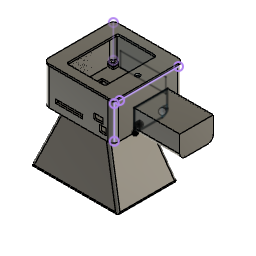
modelofinal (Autodesk Fusion 360 design; units mm, degrees)
Autodesk Fusion 360 part; units mm, degrees
(part 1 of 3)
sketch "Boceto1" plane through (0, 0, 0) normal (0, 0, 1) x (1, 0, 0)
  line L0 (0, 0) -> (95, 0)
  line L1 (95, 0) -> (95, 65)
  line L2 (95, 65) -> (0, 65)
  line L3 (0, 65) -> (0, 0)
  dimension "d1" = 95
  dimension "d2" = 65
  constraint horizontal L0
  constraint vertical L1
  constraint horizontal L2
  constraint vertical L3
  constraint coincident L0.start L3.end
  measures "d1" distance of L1.end L2.end
  measures "d2" distance of L0.start L2.end
extrude "Extruir1" add sketch "Boceto1" along normal blind 1.5 makes body 1
sketch "Boceto3" plane through (47.5, 32.5, 66.5) normal (0, 0, 1) x (1, 0, 0)
  line L0 (-47.5, 32.5) -> (-47.5, -32.5)
  line L1 (-47.5, -32.5) -> (47.5, -32.5)
  line L2 (47.5, -32.5) -> (47.5, 32.5)
  line L3 (47.5, 32.5) -> (-47.5, 32.5)
  line L4 (-22.128, 7.128) -> (-22.128, -7.128) construction
  line L5 (-22.128, -7.128) -> (22.128, -7.128) construction
  line L6 (22.128, -7.128) -> (22.128, 7.128) construction
  line L7 (22.128, 7.128) -> (-22.128, 7.128) construction
  line L8 (22.5, 20) -> (-22.5, 20)
  line L9 (-22.5, 20) -> (-22.5, -20)
  line L10 (-22.5, -20) -> (22.5, -20)
  line L11 (22.5, -20) -> (22.5, 20)
  dimension "d11" = -25.372
  dimension "d12" = 45
  dimension "d13" = 40
  dimension "d14" = 12.5
  dimension "d15" = 25
  constraint horizontal L8
  constraint vertical L9
  constraint horizontal L10
  constraint vertical L11
  measures "d12" distance of L8.start L8.end
  measures "d13" distance of L8.start L10.end
  measures "d14" distance of L3 L8
  measures "d15" distance of L0 L9
loft "Solevación1" add profiles "Boceto3" section 1 face at (31.6667, 43.3333, 1.5) section 2 contours L8 L9 L10 L11 on bodies 1 bodies 1
shell "Vaciado1" thickness 2 removed faces 1 at (40, 25.8333, 66.5) on bodies 1
extrude "Extruir2" add 1 faces at (25.7143, 26.5122, 66.5) along direction (0, 0, 1) blind 5 on bodies 1 bodies 1
sketch "Boceto4" plane through (25, 0, 0) normal (-1, 0, 0) x (0, -1, 0)
  line L0 (-52.5, 66.5) -> (-12.5, 66.5)
  line L1 (-12.5, 66.5) -> (-12.5, 71.5)
  line L2 (-12.5, 71.5) -> (-52.5, 71.5)
  line L3 (-52.5, 71.5) -> (-52.5, 66.5)
  circle A0 centre (-46.5, 69) radius 1.5
  circle A1 centre (-18.5, 69) radius 1.5
  dimension "d19" = 3
  dimension "d20" = 6
  dimension "d21" = 3
  dimension "d22" = 6
  measures "d19" diameter of A0
  measures "d20" distance of L3 A0.centre
  measures "d21" diameter of A1
  measures "d22" distance of L1 A1.centre
extrude "Extruir3" cut sketch "Boceto4" against normal blind 50 contours A0 | A1 bodies 1
sketch "Boceto5" plane through (-0.5026, 0, 0.1933) normal (-0.933346, 0, 0.358979) x (0, -1, 0)
  line L0 (-65, 1.4) -> (0, 1.4)
  line L1 (0, 1.4) -> (-12.5, 71.042)
  line L2 (-12.5, 71.042) -> (-52.5, 71.042)
  line L3 (-63.6538, 8.9) -> (-1.3462, 8.9)
  line L4 (-62.968, 1.4) -> (-61.6219, 8.9)
  line L5 (-2.032, 1.4) -> (-3.3781, 8.9)
  line L6 (-65, 1.4) -> (-52.5, 71.042)
  dimension "d27" = 2
  dimension "d28" = 2
  constraint coincident L1 L3.end
  constraint horizontal L3
  constraint coincident L0 L4.start
  constraint coincident L3 L4.end
  constraint coincident L0 L5.start
  constraint coincident L3 L5.end
  constraint parallel L4 L6
  constraint parallel L1 L5
  measures "d27" distance of L1 L5
  measures "d28" distance of L4 L6
extrude "Extruir4" cut sketch "Boceto5" against normal blind 1 contours L0 L3 L4 L5 bodies 1
fillet "Empalme1" radius 2.5 4 edges at (82.5, 6.25, 34) (12.5, 6.25, 34) (82.5, 58.75, 34) (12.5, 58.75, 34) on bodies 1
extrude "Extruir5" cut 1 faces at (1.8308, 22.7927, 3.4744) along direction (0.933346, 0, -0.358979) blind 1 on bodies 1 bodies 1
sketch "Boceto6" plane through (0, 0, 71.5) normal (0, 0, 1) x (-1, 0, 0)
  line L0 (-27.1428, -50.4634) -> (-67.8572, -50.4634)
  line L1 (-67.8572, -50.4634) -> (-67.8572, -14.5366)
  line L2 (-67.8572, -14.5366) -> (-27.1428, -14.5366)
  line L3 (-27.1428, -14.5366) -> (-27.1428, -50.4634)
  line L4 (-70, -52.5) -> (-25, -52.5)
  line L5 (-25, -52.5) -> (-25, -12.5)
  line L6 (-25, -12.5) -> (-70, -12.5)
  line L7 (-70, -12.5) -> (-70, -52.5)
sketch "Boceto7" plane through (47.5, 32.5, 71.51) normal (0, 0, 1) x (1, 0, 0)
sketch "Boceto8" plane through (0, 0, 71.5) normal (0, 0, 1) x (1, 0, 0)
sketch "Boceto9" plane through (0, 0, 71.5) normal (0, 0, 1) x (1, 0, 0)
  line L0 (27.1833, 50.4311) -> (67.8663, 50.4311)
  line L1 (67.8663, 50.4311) -> (67.8663, 14.5442)
  line L2 (67.8663, 14.5442) -> (27.1833, 14.5442)
  line L3 (27.1833, 14.5442) -> (27.1833, 50.4311)
  constraint horizontal L0
  constraint vertical L1
  constraint horizontal L2
  constraint vertical L3
ref_plane "PlanoDeObra3" through (47.5, 32.5, 71.6) normal (0, 0, 1) x (-1, 0, 0)
sketch "Boceto10" plane through (0, 0, 71.5) normal (0, 0, 1) x (-1, 0, 0)
  line L0 (-27.2, -50.4) -> (-67.7844, -50.4)
  line L1 (-67.7844, -50.4) -> (-67.7844, -14.5685)
  line L2 (-67.7844, -14.5685) -> (-27.2, -14.5685)
  line L3 (-27.2, -14.5685) -> (-27.2, -50.4)
  line L4 (-29.2, -16.5685) -> (-29.2, -48.4)
  line L5 (-29.2, -48.4) -> (-65.7844, -48.4)
  line L6 (-65.7844, -48.4) -> (-65.7844, -16.5685)
  line L7 (-65.7844, -16.5685) -> (-29.2, -16.5685)
  dimension "d37" = 2
  constraint horizontal L0
  constraint vertical L1
  constraint horizontal L2
  constraint vertical L3
extrude "Extruir6" add sketch "Boceto10" against normal blind 5 separate body makes body 2
sketch "Boceto11" plane through (0, 0, 71.5) normal (0, 0, 1) x (1, 0, 0)
sketch "Boceto12" plane through (0, 0, 71.5) normal (0, 0, 1) x (1, 0, 0)
  line L0 (90.1428, -5.0366) -> (25.1428, -5.0366)
  line L1 (20.1428, -0.0366) -> (20.1428, 64.9634)
  line L2 (25.1428, 69.9634) -> (90.1428, 69.9634)
  line L3 (95.1428, 64.9634) -> (95.1428, -0.0366)
  line L4 (65.8572, 16.5366) -> (29.1428, 16.5366)
  line L5 (29.1428, 16.5366) -> (29.1428, 48.4634)
  line L6 (29.1428, 48.4634) -> (65.8572, 48.4634)
  line L7 (65.8572, 48.4634) -> (65.8572, 16.5366)
  line L8 (27.1428, 50.4634) -> (67.8572, 50.4634)
  line L9 (27.1428, 14.5366) -> (27.1428, 50.4634)
  line L10 (67.8572, 14.5366) -> (27.1428, 14.5366)
  line L11 (67.8572, 50.4634) -> (67.8572, 14.5366)
  circle A0 centre (91.1428, 65.9634) radius 1.5
  circle A1 centre (24.1428, 65.9634) radius 1.5
  circle A2 centre (91.1428, -1.0366) radius 1.5
  arc A3 (90.1428, -5.0366) -> (95.1428, -0.0366) centre (90.1428, -0.0366) ccw
  circle A4 centre (24.1428, -2.0366) radius 1.5
  arc A5 (20.1428, -0.0366) -> (25.1428, -5.0366) centre (25.1428, -0.0366) ccw
  arc A6 (95.1428, 64.9634) -> (90.1428, 69.9634) centre (90.1428, 64.9634) ccw
  arc A7 (25.1428, 69.9634) -> (20.1428, 64.9634) centre (25.1428, 64.9634) ccw
  point P0 (95.1428, -5.0366)
  point P1 (20.1428, -5.0366)
  point P2 (20.1428, 69.9634)
  dimension "d40" = 2
  dimension "d41" = 2
  dimension "d42" = 2
  dimension "d43" = 2
  dimension "d44" = 75
  dimension "d45" = 75
  dimension "d46" = 9
  dimension "d47" = 19.5
  dimension "d48" = 3
  dimension "d49" = 4
  dimension "d50" = 4
  dimension "d51" = 3
  dimension "d52" = 4
  dimension "d53" = 4
  dimension "d54" = 5
  dimension "d55" = 4
  dimension "d56" = 4
  dimension "d57" = 3
  dimension "d58" = 3
  dimension "d59" = 3
  dimension "d60" = 4
  dimension "d61" = 5
  dimension "d62" = 5
  dimension "d63" = 5
  constraint horizontal L0
  constraint vertical L1
  constraint horizontal L2
  constraint vertical L3
  constraint horizontal L4
  constraint vertical L5
  constraint horizontal L6
  constraint vertical L7
  constraint coincident P0 L0
  constraint coincident P0 L3
  constraint tangent L0 A3
  constraint tangent L3 A3
  constraint coincident P1 L0
  constraint coincident P1 L1
  constraint tangent L0 A5
  constraint tangent L1 A5
  constraint tangent L2 A6
  constraint tangent L3 A6
  constraint coincident P2 L1
  constraint coincident P2 L2
  constraint tangent L1 A7
  constraint tangent L2 A7
  measures "d40" distance of L6 L8
  measures "d41" distance of L5 L9
  measures "d42" distance of L4 L10
  measures "d43" distance of L7 L11
  measures "d44" distance of P1 P2
  measures "d45" distance of P0 P1
  measures "d46" distance of L1 L5
  measures "d47" distance of L2 L8
  measures "d48" diameter of A0
  measures "d49" distance of L2 A0.centre
  measures "d50" distance of L3 A0.centre
  measures "d51" diameter of A2
  measures "d52" distance of L3 A2.centre
  measures "d53" distance of L0 A2.centre
  measures "d54" radius of A3
  measures "d55" distance of L2 A1.centre
  measures "d56" distance of L1 A1.centre
  measures "d57" diameter of A1
  measures "d58" diameter of A4
  measures "d59" distance of L0 A4.centre
  measures "d60" distance of L1 A4.centre
  measures "d61" radius of A5
  measures "d62" radius of A6
  measures "d63" radius of A7
extrude "Extruir7" add sketch "Boceto12" along normal blind 2 contours L0 L1 L2 L3 A3 A5 A6 A7 | L8 L9 L10 L11 bodies 2
sketch "Boceto13" plane through (0, 0, 71.5) normal (0, 0, -1) x (1, 0, 0)
  arc A0 (90.1428, -69.9634) -> (95.1428, -64.9634) centre (90.1428, -64.9634) ccw
  line L0 (95.1428, -64.9634) -> (95.1428, 0.0366)
  arc A1 (95.1428, 0.0366) -> (90.1428, 5.0366) centre (90.1428, 0.0366) ccw
  line L1 (90.1428, 5.0366) -> (25.1428, 5.0366)
  arc A2 (25.1428, 5.0366) -> (20.1428, 0.0366) centre (25.1428, 0.0366) ccw
  line L2 (20.1428, 0.0366) -> (20.1428, -64.9634)
  arc A3 (20.1428, -64.9634) -> (25.1428, -69.9634) centre (25.1428, -64.9634) ccw
  line L3 (25.1428, -69.9634) -> (90.1428, -69.9634)
  circle A4 centre (91.1428, -65.9634) radius 1.5
  circle A5 centre (24.1428, -65.9634) radius 1.5
  circle A6 centre (91.1428, 1.0366) radius 1.5
  circle A7 centre (24.1428, 2.0366) radius 1.5
  line L4 (67.7844, -14.5685) -> (67.7844, -50.4)
  line L5 (67.7844, -50.4) -> (27.2, -50.4)
  line L6 (27.2, -50.4) -> (27.2, -14.5685)
  line L7 (27.2, -14.5685) -> (67.7844, -14.5685)
  circle A8 centre (24.1428, 2.0366) radius 1.5
  circle A9 centre (91.1428, 1.0366) radius 1.5
  circle A10 centre (91.1428, -65.9634) radius 1.5
  circle A11 centre (24.1428, -65.9634) radius 1.5
  constraint concentric A7 A8
  constraint concentric A6 A9
  constraint concentric A4 A10
  constraint concentric A5 A11
extrude "Extruir8" add sketch "Boceto13" against normal blind 1 contours A4 A10 | A5 A11 | A6 A9 | A7 A8 bodies 2
sketch "Boceto14" plane through (25, 0, 0) normal (-1, 0, 0) x (0, -1, 0)
  circle A0 centre (-18.5, 69) radius 1.5
  circle A1 centre (-46.5, 69) radius 1.5
  line L0 (-12.5, 63.9895) -> (-12.5, 71.5)
  line L1 (-12.5, 71.5) -> (-52.5, 71.5)
  line L2 (-52.5, 71.5) -> (-52.5, 63.9895)
  ellipse E0 centre (-51.2935, 59.5358) end of major axis (-49.9573, 66.484) minor radius 2.5 (-50.1268, 66.5) -> (-52.5, 63.9895) ccw
  line L3 (-50.1268, 66.5) -> (-14.8732, 66.5)
  ellipse E1 centre (-13.7065, 59.5358) end of major axis (-15.0427, 66.484) minor radius 2.5 (-12.5, 63.9895) -> (-14.8732, 66.5) ccw
  circle A2 centre (-18.5, 69) radius 1.5
  circle A3 centre (-46.5, 69) radius 1.5
  constraint concentric A0 A2
  constraint concentric A1 A3
extrude "Extruir9" cut sketch "Boceto14" against normal blind 55 contours A0 A2 | A1 A3 bodies 2
sketch "Boceto15" plane through (0, 0, 73.5) normal (0, 0, 1) x (-1, 0, 0)
  circle A0 centre (-24.1428, 2.0366) radius 1.5
  circle A1 centre (-91.1428, 1.0366) radius 1.5
  circle A2 centre (-24.1428, -65.9634) radius 1.5
  line L0 (-29.1428, -48.4634) -> (-65.8572, -48.4634)
  line L1 (-65.8572, -48.4634) -> (-65.8572, -16.5366)
  line L2 (-65.8572, -16.5366) -> (-29.1428, -16.5366)
  line L3 (-29.1428, -16.5366) -> (-29.1428, -48.4634)
  circle A3 centre (-91.1428, -65.9634) radius 1.5
  arc A4 (-95.1428, -64.9634) -> (-90.1428, -69.9634) centre (-90.1428, -64.9634) ccw
  line L4 (-90.1428, -69.9634) -> (-25.1428, -69.9634)
  arc A5 (-25.1428, -69.9634) -> (-20.1428, -64.9634) centre (-25.1428, -64.9634) ccw
  line L5 (-20.1428, -64.9634) -> (-20.1428, 0.0366)
  arc A6 (-20.1428, 0.0366) -> (-25.1428, 5.0366) centre (-25.1428, 0.0366) ccw
  line L6 (-25.1428, 5.0366) -> (-90.1428, 5.0366)
  arc A7 (-90.1428, 5.0366) -> (-95.1428, 0.0366) centre (-90.1428, 0.0366) ccw
  line L7 (-95.1428, 0.0366) -> (-95.1428, -64.9634)
  line L8 (-25.1428, 5.0366) -> (-90.1428, 5.0366)
  line L9 (-95.1428, 0.0366) -> (-95.1428, -64.9634)
  line L10 (-90.1428, -69.9634) -> (-25.1428, -69.9634)
  line L11 (-20.1428, -64.9634) -> (-20.1428, 0.0366)
  arc A8 (-90.1428, 5.0366) -> (-95.1428, 0.0366) centre (-90.1428, 0.0366) ccw
  arc A9 (-20.1428, 0.0366) -> (-25.1428, 5.0366) centre (-25.1428, 0.0366) ccw
  arc A10 (-95.1428, -64.9634) -> (-90.1428, -69.9634) centre (-90.1428, -64.9634) ccw
  arc A11 (-25.1428, -69.9634) -> (-20.1428, -64.9634) centre (-25.1428, -64.9634) ccw
  line L12 (-25.1428, 4.0366) -> (-90.1428, 4.0366)
  arc A12 (-90.1428, 4.0366) -> (-94.1428, 0.0366) centre (-90.1428, 0.0366) ccw
  line L13 (-94.1428, 0.0366) -> (-94.1428, -64.9634)
  arc A13 (-94.1428, -64.9634) -> (-90.1428, -68.9634) centre (-90.1428, -64.9634) ccw
  line L14 (-90.1428, -68.9634) -> (-25.1428, -68.9634)
  arc A14 (-25.1428, -68.9634) -> (-21.1428, -64.9634) centre (-25.1428, -64.9634) ccw
  line L15 (-21.1428, -64.9634) -> (-21.1428, 0.0366)
  arc A15 (-21.1428, 0.0366) -> (-25.1428, 4.0366) centre (-25.1428, 0.0366) ccw
  line L16 (-19.1428, -64.9634) -> (-19.1428, 0.0366)
  arc A16 (-19.1428, 0.0366) -> (-25.1428, 6.0366) centre (-25.1428, 0.0366) ccw
  line L17 (-25.1428, 6.0366) -> (-90.1428, 6.0366)
  arc A17 (-90.1428, 6.0366) -> (-96.1428, 0.0366) centre (-90.1428, 0.0366) ccw
  line L18 (-96.1428, 0.0366) -> (-96.1428, -64.9634)
  arc A18 (-96.1428, -64.9634) -> (-90.1428, -70.9634) centre (-90.1428, -64.9634) ccw
  line L19 (-90.1428, -70.9634) -> (-25.1428, -70.9634)
  arc A19 (-25.1428, -70.9634) -> (-19.1428, -64.9634) centre (-25.1428, -64.9634) ccw
  point P0 (-20.1428, 5.0366)
  point P1 (-95.1428, -69.9634)
  point P2 (-20.1428, -69.9634)
  dimension "d70" = 75
  dimension "d71" = 75
  dimension "d72" = 5
  dimension "d73" = 5
  dimension "d74" = 5
  dimension "d75" = -1
  dimension "d76" = 1
  constraint horizontal L8
  constraint vertical L9
  constraint horizontal L10
  constraint vertical L11
  constraint coincident L7 P1
  constraint coincident L6 P0
  constraint tangent L8 A8
  constraint tangent L9 A8
  constraint coincident P0 L8
  constraint coincident P0 L11
  constraint tangent L8 A9
  constraint tangent L11 A9
  constraint equal A8 A9
  constraint coincident P1 L9
  constraint coincident P1 L10
  constraint tangent L9 A10
  constraint tangent L10 A10
  constraint coincident P2 L10
  constraint coincident P2 L11
  constraint tangent L10 A11
  constraint tangent L11 A11
  measures "d70" distance of P0 P2
  measures "d71" distance of P1 P2
  measures "d72" radius of A8
  measures "d73" radius of A10
  measures "d74" radius of A11
ref_plane "PlanoDeObra4" through (57.6428, 32.4634, 74.5) normal (0, 0, 1) x (1, 0, 0)
sketch "Boceto18" plane through (0, 0, 74.5) normal (0, 0, 1) x (1, 0, 0)
  line L0 (25, 70) -> (90, 70)
  line L1 (95, 65) -> (95, 0)
  line L2 (90, -5) -> (25, -5)
  line L3 (20, 0) -> (20, 65)
  arc A0 (25, 70) -> (20, 65) centre (25, 65) ccw
  arc A1 (95, 65) -> (90, 70) centre (90, 65) ccw
  arc A2 (90, -5) -> (95, 0) centre (90, 0) ccw
  arc A3 (20, 0) -> (25, -5) centre (25, 0) ccw
  arc A4 (90, -4) -> (94, 0) centre (90, 0) ccw
  line L4 (94, 65) -> (94, 0)
  arc A5 (94, 65) -> (90, 69) centre (90, 65) ccw
  line L5 (25, 69) -> (90, 69)
  arc A6 (25, 69) -> (21, 65) centre (25, 65) ccw
  line L6 (21, 0) -> (21, 65)
  arc A7 (21, 0) -> (25, -4) centre (25, 0) ccw
  line L7 (90, -4) -> (25, -4)
  arc A8 (90, -6) -> (96, 0) centre (90, 0) ccw
  line L8 (96, 65) -> (96, 0)
  arc A9 (96, 65) -> (90, 71) centre (90, 65) ccw
  line L9 (25, 71) -> (90, 71)
  arc A10 (25, 71) -> (19, 65) centre (25, 65) ccw
  line L10 (19, 0) -> (19, 65)
  arc A11 (19, 0) -> (25, -6) centre (25, 0) ccw
  line L11 (90, -6) -> (25, -6)
  dimension "d80" = 5
  dimension "d81" = 1
  dimension "d82" = -1
  constraint horizontal L0
  constraint vertical L1
  constraint horizontal L2
  constraint vertical L3
  constraint tangent L0 A0
  constraint tangent L3 A0
  constraint tangent L0 A1
  constraint tangent L1 A1
  constraint equal A0 A1
  constraint tangent L1 A2
  constraint tangent L2 A2
  constraint equal A0 A2
  constraint tangent L2 A3
  constraint tangent L3 A3
  constraint equal A0 A3
  measures "d80" radius of A0
extrude "Extruir11" add sketch "Boceto18" along normal blind 35 separate body contours L0 L1 L2 L3 A0 A1 A2 A3 | A8 L8 A9 L9 A10 L10 A11 L11 makes body 3
sketch "Boceto19" plane through (0, 0, 109.5) normal (0, 0, 1) x (-1, 0, 0)
  arc A0 (-94, -65) -> (-90, -69) centre (-90, -65) ccw
  line L0 (-94, -65) -> (-94, 0)
  arc A1 (-90, 4) -> (-94, 0) centre (-90, 0) ccw
  line L1 (-90, 4) -> (-25, 4)
  arc A2 (-21, 0) -> (-25, 4) centre (-25, 0) ccw
  line L2 (-21, 0) -> (-21, -65)
  arc A3 (-25, -69) -> (-21, -65) centre (-25, -65) ccw
  line L3 (-25, -69) -> (-90, -69)
  arc A4 (-96, -65) -> (-90, -71) centre (-90, -65) ccw
  line L4 (-90, -71) -> (-25, -71)
  arc A5 (-25, -71) -> (-19, -65) centre (-25, -65) ccw
  line L5 (-19, -65) -> (-19, 0)
  arc A6 (-19, 0) -> (-25, 6) centre (-25, 0) ccw
  line L6 (-25, 6) -> (-90, 6)
  arc A7 (-90, 6) -> (-96, 0) centre (-90, 0) ccw
  line L7 (-96, 0) -> (-96, -65)
  line L8 (-91, 6) -> (-24, 6)
  line L9 (-19, 1) -> (-19, -66)
  line L10 (-24, -71) -> (-91, -71)
  line L11 (-96, -66) -> (-96, 1)
  arc A8 (-96, -66) -> (-91, -71) centre (-91, -66) ccw
  arc A9 (-24, -71) -> (-19, -66) centre (-24, -66) ccw
  arc A10 (-19, 1) -> (-24, 6) centre (-24, 1) ccw
  arc A11 (-91, 6) -> (-96, 1) centre (-91, 1) ccw
  arc A12 (-24, -70) -> (-20, -66) centre (-24, -66) ccw
  line L12 (-20, 1) -> (-20, -66)
  arc A13 (-20, 1) -> (-24, 5) centre (-24, 1) ccw
  line L13 (-91, 5) -> (-24, 5)
  arc A14 (-91, 5) -> (-95, 1) centre (-91, 1) ccw
  line L14 (-95, -66) -> (-95, 1)
  arc A15 (-95, -66) -> (-91, -70) centre (-91, -66) ccw
  line L15 (-24, -70) -> (-91, -70)
  dimension "d85" = 5
  dimension "d86" = 1
  constraint horizontal L8
  constraint vertical L9
  constraint horizontal L10
  constraint vertical L11
  constraint tangent L10 A8
  constraint tangent L11 A8
  constraint tangent L9 A9
  constraint tangent L10 A9
  constraint equal A8 A9
  constraint tangent L8 A10
  constraint tangent L9 A10
  constraint equal A8 A10
  constraint tangent L8 A11
  constraint tangent L11 A11
  constraint equal A8 A11
  measures "d85" radius of A8
extrude "Extruir12" add sketch "Boceto19" along normal blind 1 contours A4 L4 A5 L5 A6 L6 A7 L7 L8 L9 L10 L11 bodies 3
ref_plane "PlanoDeObra5" through (57.5, 32.5, 110.6) normal (0, 0, 1) x (-1, 0, 0)
sketch "Boceto20" plane through (0, 0, 110.6) normal (0, 0, 1) x (1, 0, 0)
  line L0 (91, -6) -> (24, -6)
  line L1 (19, -1) -> (19, 66)
  line L2 (24, 71) -> (91, 71)
  line L3 (96, 66) -> (96, -1)
  arc A0 (96, 66) -> (91, 71) centre (91, 66) ccw
  arc A1 (24, 71) -> (19, 66) centre (24, 66) ccw
  arc A2 (19, -1) -> (24, -6) centre (24, -1) ccw
  arc A3 (91, -6) -> (96, -1) centre (91, -1) ccw
  arc A4 (24, 69) -> (21, 66) centre (24, 66) ccw
  line L4 (21, -1) -> (21, 66)
  arc A5 (21, -1) -> (24, -4) centre (24, -1) ccw
  line L5 (91, -4) -> (24, -4)
  arc A6 (91, -4) -> (94, -1) centre (91, -1) ccw
  line L6 (94, 66) -> (94, -1)
  arc A7 (94, 66) -> (91, 69) centre (91, 66) ccw
  line L7 (24, 69) -> (91, 69)
  dimension "d90" = 5
  dimension "d91" = 2
  constraint horizontal L0
  constraint vertical L1
  constraint horizontal L2
  constraint vertical L3
  constraint tangent L2 A0
  constraint tangent L3 A0
  constraint tangent L1 A1
  constraint tangent L2 A1
  constraint equal A0 A1
  constraint tangent L0 A2
  constraint tangent L1 A2
  constraint equal A0 A2
  constraint tangent L0 A3
  constraint tangent L3 A3
  constraint equal A0 A3
  measures "d90" radius of A0
extrude "Extruir13" add sketch "Boceto20" along normal blind 2 separate body contours L0 L1 L2 L3 A0 A1 A2 A3 | A4 L4 A5 L5 A6 L6 A7 L7 makes body 4
sketch "Boceto21" plane through (0, 0, 110.6) normal (0, 0, -1) x (1, 0, 0)
  arc A0 (24, 6) -> (19, 1) centre (24, 1) ccw
  line L0 (19, 1) -> (19, -66)
  arc A1 (19, -66) -> (24, -71) centre (24, -66) ccw
  line L1 (24, -71) -> (91, -71)
  arc A2 (91, -71) -> (96, -66) centre (91, -66) ccw
  line L2 (96, -66) -> (96, 1)
  arc A3 (96, 1) -> (91, 6) centre (91, 1) ccw
  line L3 (91, 6) -> (24, 6)
  line L4 (24, -70) -> (91, -70)
  arc A4 (91, -70) -> (95, -66) centre (91, -66) ccw
  line L5 (95, -66) -> (95, 1)
  arc A5 (95, 1) -> (91, 5) centre (91, 1) ccw
  line L6 (91, 5) -> (24, 5)
  arc A6 (24, 5) -> (20, 1) centre (24, 1) ccw
  line L7 (20, 1) -> (20, -66)
  arc A7 (20, -66) -> (24, -70) centre (24, -66) ccw
  line L8 (91, -70) -> (24, -70)
  line L9 (20, -66) -> (20, 1)
  line L10 (24, 5) -> (91, 5)
  line L11 (95, 1) -> (95, -66)
  arc A8 (91, -70) -> (95, -66) centre (91, -66) ccw
  arc A9 (95, 1) -> (91, 5) centre (91, 1) ccw
  arc A10 (24, 5) -> (20, 1) centre (24, 1) ccw
  arc A11 (20, -66) -> (24, -70) centre (24, -66) ccw
  arc A12 (24, 4) -> (21, 1) centre (24, 1) ccw
  line L12 (21, -66) -> (21, 1)
  arc A13 (21, -66) -> (24, -69) centre (24, -66) ccw
  line L13 (91, -69) -> (24, -69)
  arc A14 (91, -69) -> (94, -66) centre (91, -66) ccw
  line L14 (94, 1) -> (94, -66)
  arc A15 (94, 1) -> (91, 4) centre (91, 1) ccw
  line L15 (24, 4) -> (91, 4)
  dimension "d94" = -1
  dimension "d95" = 4
  dimension "d96" = 1
  constraint horizontal L8
  constraint vertical L9
  constraint horizontal L10
  constraint vertical L11
  constraint tangent L8 A8
  constraint tangent L11 A8
  constraint tangent L10 A9
  constraint tangent L11 A9
  constraint equal A8 A9
  constraint tangent L9 A10
  constraint tangent L10 A10
  constraint equal A8 A10
  constraint tangent L8 A11
  constraint tangent L9 A11
  constraint equal A8 A11
  measures "d95" radius of A8
extrude "Extruir14" add sketch "Boceto21" along normal blind 1 contours L4 A4 L5 A5 L6 A6 L7 A7 L8 L9 L10 L11 A8 A9 A10 A11 bodies 4
sketch "Boceto22" plane through (0, 0, 112.6) normal (0, 0, 1) x (-1, 0, 0)
  arc A0 (-19, 1) -> (-24, 6) centre (-24, 1) ccw
  line L0 (-24, 6) -> (-91, 6)
  arc A1 (-91, 6) -> (-96, 1) centre (-91, 1) ccw
  line L1 (-96, 1) -> (-96, -66)
  arc A2 (-96, -66) -> (-91, -71) centre (-91, -66) ccw
  line L2 (-91, -71) -> (-24, -71)
  arc A3 (-24, -71) -> (-19, -66) centre (-24, -66) ccw
  line L3 (-19, -66) -> (-19, 1)
  line L4 (-36, -4) -> (-75, -4)
  line L5 (-77, -6) -> (-77, -59)
  line L6 (-75, -61) -> (-36, -61)
  line L7 (-34, -59) -> (-34, -6)
  circle A4 centre (-85, -32) radius 2.5
  arc A5 (-34, -6) -> (-36, -4) centre (-36, -6) ccw
  arc A6 (-36, -61) -> (-34, -59) centre (-36, -59) ccw
  arc A7 (-77, -59) -> (-75, -61) centre (-75, -59) ccw
  arc A8 (-75, -4) -> (-77, -6) centre (-75, -6) ccw
  point P0 (-34, -4)
  point P1 (-34, -61)
  dimension "d99" = 57
  dimension "d100" = 10
  dimension "d101" = 43
  dimension "d102" = 15
  dimension "d103" = 5
  dimension "d104" = 38
  dimension "d105" = 2
  dimension "d106" = 2
  dimension "d107" = 2
  dimension "d108" = 2
  constraint horizontal L4
  constraint vertical L5
  constraint horizontal L6
  constraint vertical L7
  constraint coincident P0 L4
  constraint coincident P0 L7
  constraint tangent L4 A5
  constraint tangent L7 A5
  constraint coincident P1 L6
  constraint coincident P1 L7
  constraint tangent L6 A6
  constraint tangent L7 A6
  constraint tangent L5 A7
  constraint tangent L6 A7
  constraint tangent L4 A8
  constraint tangent L5 A8
  measures "d99" distance of P0 P1
  measures "d100" distance of L0 L4
  measures "d101" distance of L5 L7
  measures "d102" distance of L3 L7
  measures "d103" diameter of A4
  measures "d104" distance of L0 A4.centre
  measures "d105" radius of A5
  measures "d106" radius of A6
  measures "d107" radius of A7
  measures "d108" radius of A8
sketch "Boceto23" plane through (19, 0, 0) normal (-1, 0, 0) x (0, -1, 0)
  line L0 (-65, 74.5) -> (0, 74.5)
  line L1 (0, 74.5) -> (0, 110.5)
  line L2 (0, 110.5) -> (-65, 110.5)
  line L3 (-65, 110.5) -> (-65, 74.5)
ref_plane "PlanoDeObra6" through (18, 32.5, 92.5) normal (-1, 0, 0) x (0, -1, 0)
sketch "Boceto24" plane through (18, 0, 0) normal (-1, 0, 0) x (0, -1, 0)
  line L0 (-53, 111) -> (-16.5822, 111)
  line L1 (-16.5822, 111) -> (-16.5822, 74.5822)
  line L2 (-16.5822, 74.5822) -> (-53, 74.5822)
  line L3 (-53, 74.5822) -> (-53, 111)
  line L4 (-45.7805, 91.3685) -> (-40.6236, 91.3685)
  line L5 (-40.6236, 91.3685) -> (-40.5881, 91.333)
  line L6 (-40.5881, 91.333) -> (-40.4814, 90.515)
  line L7 (-40.4814, 90.515) -> (-40.4814, 90.3016)
  line L8 (-40.4814, 90.3016) -> (-41.1215, 89.8393)
  line L9 (-41.1215, 89.8393) -> (-41.7973, 89.3769)
  line L10 (-41.7973, 89.3769) -> (-41.904, 89.4125)
  line L11 (-41.904, 89.4125) -> (-42.1173, 89.697)
  line L12 (-42.1173, 89.697) -> (-42.4374, 89.9104)
  line L13 (-42.4374, 89.9104) -> (-42.7219, 89.9815)
  line L14 (-42.7219, 89.9815) -> (-43.1843, 89.9815)
  line L15 (-43.1843, 89.9815) -> (-43.5043, 89.8748)
  line L16 (-43.5043, 89.8748) -> (-43.8244, 89.6614)
  line L17 (-43.8244, 89.6614) -> (-44.0734, 89.3058)
  line L18 (-44.0734, 89.3058) -> (-44.1801, 88.9146)
  line L19 (-44.1801, 88.9146) -> (-44.1801, 88.5945)
  line L20 (-44.1801, 88.5945) -> (-44.0734, 88.2389)
  line L21 (-44.0734, 88.2389) -> (-43.86, 87.9188)
  line L22 (-43.86, 87.9188) -> (-43.611, 87.7054)
  line L23 (-43.611, 87.7054) -> (-43.2198, 87.5632)
  line L24 (-43.2198, 87.5632) -> (-42.6508, 87.5632)
  line L25 (-42.6508, 87.5632) -> (-42.2952, 87.7054)
  line L26 (-42.2952, 87.7054) -> (-41.9751, 87.9899)
  line L27 (-41.9751, 87.9899) -> (-41.7617, 88.4167)
  line L28 (-41.7617, 88.4167) -> (-41.6906, 88.6656)
  line L29 (-41.6906, 88.6656) -> (-41.1571, 89.0569)
  line L30 (-41.1571, 89.0569) -> (-40.5525, 89.4836)
  line L31 (-40.5525, 89.4836) -> (-40.3391, 89.6259)
  line L32 (-40.3391, 89.6259) -> (-40.2324, 89.6259)
  line L33 (-40.2324, 89.6259) -> (-39.8412, 88.7723)
  line L34 (-39.8412, 88.7723) -> (-39.6634, 88.4878)
  line L35 (-39.6634, 88.4878) -> (-39.7345, 88.3456)
  line L36 (-39.7345, 88.3456) -> (-40.1613, 87.9188)
  line L37 (-40.1613, 87.9188) -> (-40.4458, 87.6698)
  line L38 (-40.4458, 87.6698) -> (-40.9437, 87.172)
  line L39 (-40.9437, 87.172) -> (-41.2282, 86.923)
  line L40 (-41.2282, 86.923) -> (-41.3705, 86.9586)
  line L41 (-41.3705, 86.9586) -> (-41.655, 87.1364)
  line L42 (-41.655, 87.1364) -> (-42.0818, 87.2075)
  line L43 (-42.0818, 87.2075) -> (-42.4019, 87.1364)
  line L44 (-42.4019, 87.1364) -> (-42.6864, 86.9941)
  line L45 (-42.6864, 86.9941) -> (-42.8998, 86.7452)
  line L46 (-42.8998, 86.7452) -> (-43.042, 86.3895)
  line L47 (-43.042, 86.3895) -> (-43.042, 85.9628)
  line L48 (-43.042, 85.9628) -> (-42.9353, 85.6783)
  line L49 (-42.9353, 85.6783) -> (-42.6508, 85.3582)
  line L50 (-42.6508, 85.3582) -> (-42.3307, 85.2159)
  line L51 (-42.3307, 85.2159) -> (-42.1885, 85.1804)
  line L52 (-42.1885, 85.1804) -> (-41.8328, 85.1804)
  line L53 (-41.8328, 85.1804) -> (-41.4772, 85.287)
  line L54 (-41.4772, 85.287) -> (-41.1927, 85.536)
  line L55 (-41.1927, 85.536) -> (-41.0504, 85.7849)
  line L56 (-41.0504, 85.7849) -> (-40.9793, 86.2473)
  line L57 (-40.9793, 86.2473) -> (-40.5525, 86.6385)
  line L58 (-40.5525, 86.6385) -> (-39.8412, 87.3498)
  line L59 (-39.8412, 87.3498) -> (-39.2722, 87.8477)
  line L60 (-39.2722, 87.8477) -> (-39.1299, 87.7765)
  line L61 (-39.1299, 87.7765) -> (-38.5253, 87.172)
  line L62 (-38.5253, 87.172) -> (-38.4187, 87.1008)
  line L63 (-38.4187, 87.1008) -> (-38.4187, 86.9941)
  line L64 (-38.4187, 86.9941) -> (-39.2722, 86.1406)
  line L65 (-39.2722, 86.1406) -> (-39.3433, 86.1406)
  line L66 (-39.3433, 86.1406) -> (-39.3433, 86.0695)
  line L67 (-39.3433, 86.0695) -> (-39.6278, 85.8205)
  line L68 (-39.6278, 85.8205) -> (-39.7701, 85.6427)
  line L69 (-39.7701, 85.6427) -> (-39.8412, 85.6427)
  line L70 (-39.8412, 85.6427) -> (-39.8412, 85.5716)
  line L71 (-39.8412, 85.5716) -> (-39.9124, 85.5716)
  line L72 (-39.9124, 85.5716) -> (-39.9835, 85.4293)
  line L73 (-39.9835, 85.4293) -> (-40.4458, 85.0025)
  line L74 (-40.4458, 85.0025) -> (-40.9437, 84.4691)
  line L75 (-40.9437, 84.4691) -> (-41.2282, 84.2201)
  line L76 (-41.2282, 84.2201) -> (-41.5127, 83.9356)
  line L77 (-41.5127, 83.9356) -> (-41.5839, 83.7933)
  line L78 (-41.5839, 83.7933) -> (-41.5483, 83.5444)
  line L79 (-41.5483, 83.5444) -> (-41.3705, 83.4021)
  line L80 (-41.3705, 83.4021) -> (-41.1215, 83.4021)
  line L81 (-41.1215, 83.4021) -> (-40.837, 83.6511)
  line L82 (-40.837, 83.6511) -> (-37.8496, 86.6385)
  line L83 (-37.8496, 86.6385) -> (-37.6718, 86.6029)
  line L84 (-37.6718, 86.6029) -> (-36.8183, 86.1762)
  line L85 (-36.8183, 86.1762) -> (-36.8894, 85.9983)
  line L86 (-36.8894, 85.9983) -> (-37.1383, 85.7138)
  line L87 (-37.1383, 85.7138) -> (-38.7743, 84.0779)
  line L88 (-38.7743, 84.0779) -> (-39.3078, 83.9712)
  line L89 (-39.3078, 83.9712) -> (-39.6278, 83.7578)
  line L90 (-39.6278, 83.7578) -> (-39.8412, 83.4733)
  line L91 (-39.8412, 83.4733) -> (-39.9479, 83.0465)
  line L92 (-39.9479, 83.0465) -> (-39.8768, 82.6197)
  line L93 (-39.8768, 82.6197) -> (-39.699, 82.2996)
  line L94 (-39.699, 82.2996) -> (-39.45, 82.0863)
  line L95 (-39.45, 82.0863) -> (-39.1299, 81.9796)
  line L96 (-39.1299, 81.9796) -> (-38.6676, 81.9796)
  line L97 (-38.6676, 81.9796) -> (-38.312, 82.1218)
  line L98 (-38.312, 82.1218) -> (-38.063, 82.3708)
  line L99 (-38.063, 82.3708) -> (-37.9208, 82.6553)
  line L100 (-37.9208, 82.6553) -> (-37.8852, 82.762)
  line L101 (-37.8852, 82.762) -> (-37.8852, 83.1888)
  line L102 (-37.8852, 83.1888) -> (-38.0274, 83.5444)
  line L103 (-38.0274, 83.5444) -> (-38.1341, 83.6867)
  line L104 (-38.1341, 83.6867) -> (-38.0986, 83.8289)
  line L105 (-38.0986, 83.8289) -> (-36.8894, 85.0381)
  line L106 (-36.8894, 85.0381) -> (-36.8183, 85.0381)
  line L107 (-36.8183, 85.0381) -> (-36.8183, 81.6595)
  line L108 (-36.8183, 81.6595) -> (-36.7116, 81.4461)
  line L109 (-36.7116, 81.4461) -> (-36.6404, 81.4105)
  line L110 (-36.6404, 81.4105) -> (-36.3915, 81.4105)
  line L111 (-36.3915, 81.4105) -> (-36.2137, 81.5884)
  line L112 (-36.2137, 81.5884) -> (-36.1781, 85.9983)
  line L113 (-36.1781, 85.9983) -> (-35.2534, 85.8561)
  line L114 (-35.2534, 85.8561) -> (-34.9689, 85.8205)
  line L115 (-34.9689, 85.8205) -> (-34.9334, 85.7849)
  line L116 (-34.9334, 85.7849) -> (-34.8978, 81.9796)
  line L117 (-34.8978, 81.9796) -> (-34.7911, 81.8017)
  line L118 (-34.7911, 81.8017) -> (-34.6844, 81.7306)
  line L119 (-34.6844, 81.7306) -> (-34.4355, 81.7662)
  line L120 (-34.4355, 81.7662) -> (-34.3288, 81.8729)
  line L121 (-34.3288, 81.8729) -> (-34.2932, 81.944)
  line L122 (-34.2932, 81.944) -> (-34.2576, 85.8205)
  line L123 (-34.2576, 85.8205) -> (-33.3685, 85.9272)
  line L124 (-33.3685, 85.9272) -> (-33.0485, 85.9628)
  line L125 (-33.0485, 85.9628) -> (-33.0129, 81.6595)
  line L126 (-33.0129, 81.6595) -> (-32.9062, 81.4461)
  line L127 (-32.9062, 81.4461) -> (-32.8351, 81.4105)
  line L128 (-32.8351, 81.4105) -> (-32.5506, 81.4105)
  line L129 (-32.5506, 81.4105) -> (-32.4439, 81.4461)
  line L130 (-32.4439, 81.4461) -> (-32.4083, 81.5528)
  line L131 (-32.4083, 81.5528) -> (-32.3727, 85.0381)
  line L132 (-32.3727, 85.0381) -> (-32.1949, 84.9314)
  line L133 (-32.1949, 84.9314) -> (-31.128, 83.8645)
  line L134 (-31.128, 83.8645) -> (-31.0924, 83.6867)
  line L135 (-31.0924, 83.6867) -> (-31.2702, 83.4021)
  line L136 (-31.2702, 83.4021) -> (-31.3414, 83.0821)
  line L137 (-31.3414, 83.0821) -> (-31.3058, 82.6909)
  line L138 (-31.3058, 82.6909) -> (-31.1635, 82.4063)
  line L139 (-31.1635, 82.4063) -> (-30.9857, 82.193)
  line L140 (-30.9857, 82.193) -> (-30.6656, 82.0151)
  line L141 (-30.6656, 82.0151) -> (-30.5234, 81.9796)
  line L142 (-30.5234, 81.9796) -> (-30.0966, 81.9796)
  line L143 (-30.0966, 81.9796) -> (-29.7765, 82.0863)
  line L144 (-29.7765, 82.0863) -> (-29.4565, 82.3708)
  line L145 (-29.4565, 82.3708) -> (-29.3142, 82.6909)
  line L146 (-29.3142, 82.6909) -> (-29.2786, 82.8331)
  line L147 (-29.2786, 82.8331) -> (-29.2786, 83.1176)
  line L148 (-29.2786, 83.1176) -> (-29.3853, 83.4733)
  line L149 (-29.3853, 83.4733) -> (-29.5987, 83.7578)
  line L150 (-29.5987, 83.7578) -> (-29.9188, 83.9712)
  line L151 (-29.9188, 83.9712) -> (-30.3456, 84.0423)
  line L152 (-30.3456, 84.0423) -> (-30.559, 84.1846)
  line L153 (-30.559, 84.1846) -> (-30.8079, 84.4691)
  line L154 (-30.8079, 84.4691) -> (-32.3727, 86.0339)
  line L155 (-32.3727, 86.0339) -> (-32.3727, 86.1762)
  line L156 (-32.3727, 86.1762) -> (-31.6259, 86.5318)
  line L157 (-31.6259, 86.5318) -> (-31.4481, 86.6385)
  line L158 (-31.4481, 86.6385) -> (-31.3058, 86.6029)
  line L159 (-31.3058, 86.6029) -> (-28.1406, 83.4377)
  line L160 (-28.1406, 83.4377) -> (-28.0695, 83.4021)
  line L161 (-28.0695, 83.4021) -> (-27.8205, 83.4021)
  line L162 (-27.8205, 83.4021) -> (-27.6783, 83.4733)
  line L163 (-27.6783, 83.4733) -> (-27.6071, 83.6155)
  line L164 (-27.6071, 83.6155) -> (-27.6071, 83.8289)
  line L165 (-27.6071, 83.8289) -> (-27.9272, 84.1846)
  line L166 (-27.9272, 84.1846) -> (-28.7807, 85.0381)
  line L167 (-28.7807, 85.0381) -> (-29.0653, 85.287)
  line L168 (-29.0653, 85.287) -> (-30.8079, 87.0297)
  line L169 (-30.8079, 87.0297) -> (-30.5945, 87.2786)
  line L170 (-30.5945, 87.2786) -> (-30.2744, 87.5632)
  line L171 (-30.2744, 87.5632) -> (-30.0611, 87.8121)
  line L172 (-30.0611, 87.8121) -> (-29.9188, 87.7765)
  line L173 (-29.9188, 87.7765) -> (-29.3853, 87.2786)
  line L174 (-29.3853, 87.2786) -> (-28.7807, 86.7096)
  line L175 (-28.7807, 86.7096) -> (-28.4251, 86.3895)
  line L176 (-28.4251, 86.3895) -> (-28.2473, 86.2473)
  line L177 (-28.2473, 86.2473) -> (-28.1406, 85.7849)
  line L178 (-28.1406, 85.7849) -> (-27.9272, 85.4649)
  line L179 (-27.9272, 85.4649) -> (-27.6071, 85.2515)
  line L180 (-27.6071, 85.2515) -> (-27.3582, 85.1804)
  line L181 (-27.3582, 85.1804) -> (-26.967, 85.1804)
  line L182 (-26.967, 85.1804) -> (-26.6113, 85.3226)
  line L183 (-26.6113, 85.3226) -> (-26.3268, 85.5716)
  line L184 (-26.3268, 85.5716) -> (-26.1846, 85.8561)
  line L185 (-26.1846, 85.8561) -> (-26.149, 85.9983)
  line L186 (-26.149, 85.9983) -> (-26.149, 86.354)
  line L187 (-26.149, 86.354) -> (-26.2557, 86.6741)
  line L188 (-26.2557, 86.6741) -> (-26.4691, 86.923)
  line L189 (-26.4691, 86.923) -> (-26.4691, 86.9941)
  line L190 (-26.4691, 86.9941) -> (-26.6469, 87.0653)
  line L191 (-26.6469, 87.0653) -> (-26.8603, 87.172)
  line L192 (-26.8603, 87.172) -> (-27.2515, 87.2075)
  line L193 (-27.2515, 87.2075) -> (-27.6783, 87.1008)
  line L194 (-27.6783, 87.1008) -> (-27.9272, 86.8874)
  line L195 (-27.9272, 86.8874) -> (-28.0695, 86.9586)
  line L196 (-28.0695, 86.9586) -> (-28.6029, 87.4565)
  line L197 (-28.6029, 87.4565) -> (-28.923, 87.7765)
  line L198 (-28.923, 87.7765) -> (-29.2075, 88.0255)
  line L199 (-29.2075, 88.0255) -> (-29.5632, 88.3811)
  line L200 (-29.5632, 88.3811) -> (-29.5276, 88.5234)
  line L201 (-29.5276, 88.5234) -> (-29.2075, 89.0924)
  line L202 (-29.2075, 89.0924) -> (-28.9941, 89.5548)
  line L203 (-28.9941, 89.5548) -> (-28.8874, 89.5548)
  line L204 (-28.8874, 89.5548) -> (-27.7138, 88.7723)
  line L205 (-27.7138, 88.7723) -> (-27.5716, 88.6656)
  line L206 (-27.5716, 88.6656) -> (-27.4649, 88.2744)
  line L207 (-27.4649, 88.2744) -> (-27.2515, 87.9188)
  line L208 (-27.2515, 87.9188) -> (-26.9314, 87.6698)
  line L209 (-26.9314, 87.6698) -> (-26.6113, 87.5632)
  line L210 (-26.6113, 87.5632) -> (-26.0423, 87.5632)
  line L211 (-26.0423, 87.5632) -> (-25.6511, 87.7054)
  line L212 (-25.6511, 87.7054) -> (-25.4021, 87.9188)
  line L213 (-25.4021, 87.9188) -> (-25.1888, 88.2744)
  line L214 (-25.1888, 88.2744) -> (-25.1176, 88.4878)
  line L215 (-25.1176, 88.4878) -> (-25.1176, 89.0569)
  line L216 (-25.1176, 89.0569) -> (-25.2599, 89.4125)
  line L217 (-25.2599, 89.4125) -> (-25.58, 89.7681)
  line L218 (-25.58, 89.7681) -> (-25.9356, 89.946)
  line L219 (-25.9356, 89.946) -> (-26.0779, 89.9815)
  line L220 (-26.0779, 89.9815) -> (-26.6113, 89.9815)
  line L221 (-26.6113, 89.9815) -> (-27.0381, 89.8037)
  line L222 (-27.0381, 89.8037) -> (-27.287, 89.5903)
  line L223 (-27.287, 89.5903) -> (-27.4293, 89.3769)
  line L224 (-27.4293, 89.3769) -> (-27.8561, 89.5903)
  line L225 (-27.8561, 89.5903) -> (-28.6029, 90.0882)
  line L226 (-28.6029, 90.0882) -> (-28.7807, 90.2305)
  line L227 (-28.7807, 90.2305) -> (-28.6741, 90.9418)
  line L228 (-28.6741, 90.9418) -> (-28.6385, 91.333)
  line L229 (-28.6385, 91.333) -> (-28.6029, 91.3685)
  line L230 (-28.6029, 91.3685) -> (-23.4105, 91.3685)
  line L231 (-23.4105, 91.3685) -> (-23.375, 91.2618)
  line L232 (-23.375, 91.2618) -> (-23.4817, 90.3727)
  line L233 (-23.4817, 90.3727) -> (-23.7306, 89.0924)
  line L234 (-23.7306, 89.0924) -> (-24.0863, 87.8832)
  line L235 (-24.0863, 87.8832) -> (-24.4419, 86.9586)
  line L236 (-24.4419, 86.9586) -> (-24.762, 86.2473)
  line L237 (-24.762, 86.2473) -> (-25.1888, 85.3937)
  line L238 (-25.1888, 85.3937) -> (-25.6155, 84.6825)
  line L239 (-25.6155, 84.6825) -> (-26.0779, 84.0067)
  line L240 (-26.0779, 84.0067) -> (-26.5046, 83.4377)
  line L241 (-26.5046, 83.4377) -> (-26.8958, 82.9754)
  line L242 (-26.8958, 82.9754) -> (-27.2159, 82.5842)
  line L243 (-27.2159, 82.5842) -> (-27.6071, 82.193)
  line L244 (-27.6071, 82.193) -> (-27.8561, 81.9084)
  line L245 (-27.8561, 81.9084) -> (-28.3895, 81.4105)
  line L246 (-28.3895, 81.4105) -> (-28.4962, 81.2683)
  line L247 (-28.4962, 81.2683) -> (-26.6113, 81.1972)
  line L248 (-26.6113, 81.1972) -> (-24.9398, 81.0905)
  line L249 (-24.9398, 81.0905) -> (-24.2285, 81.0193)
  line L250 (-24.2285, 81.0193) -> (-23.5528, 80.9126)
  line L251 (-23.5528, 80.9126) -> (-23.375, 80.8059)
  line L252 (-23.375, 80.8059) -> (-23.375, 80.7348)
  line L253 (-23.375, 80.7348) -> (-23.6239, 80.6281)
  line L254 (-23.6239, 80.6281) -> (-24.513, 80.5214)
  line L255 (-24.513, 80.5214) -> (-26.3624, 80.4147)
  line L256 (-26.3624, 80.4147) -> (-28.1762, 80.3436)
  line L257 (-28.1762, 80.3436) -> (-31.0569, 80.2725)
  line L258 (-31.0569, 80.2725) -> (-38.2053, 80.2725)
  line L259 (-38.2053, 80.2725) -> (-41.1215, 80.3436)
  line L260 (-41.1215, 80.3436) -> (-43.3977, 80.4503)
  line L261 (-43.3977, 80.4503) -> (-44.8202, 80.557)
  line L262 (-44.8202, 80.557) -> (-45.3181, 80.6281)
  line L263 (-45.3181, 80.6281) -> (-45.5671, 80.7348)
  line L264 (-45.5671, 80.7348) -> (-45.5315, 80.8771)
  line L265 (-45.5315, 80.8771) -> (-45.1047, 80.9838)
  line L266 (-45.1047, 80.9838) -> (-43.6822, 81.126)
  line L267 (-43.6822, 81.126) -> (-41.7973, 81.2327)
  line L268 (-41.7973, 81.2327) -> (-40.6948, 81.2683)
  line L269 (-40.6948, 81.2683) -> (-40.9082, 81.5172)
  line L270 (-40.9082, 81.5172) -> (-41.1571, 81.7306)
  line L271 (-41.1571, 81.7306) -> (-41.1571, 81.8017)
  line L272 (-41.1571, 81.8017) -> (-41.2994, 81.8729)
  line L273 (-41.2994, 81.8729) -> (-41.6906, 82.2641)
  line L274 (-41.6906, 82.2641) -> (-41.9395, 82.5486)
  line L275 (-41.9395, 82.5486) -> (-42.2952, 82.9398)
  line L276 (-42.2952, 82.9398) -> (-42.6864, 83.4377)
  line L277 (-42.6864, 83.4377) -> (-43.1487, 84.0423)
  line L278 (-43.1487, 84.0423) -> (-43.5043, 84.5758)
  line L279 (-43.5043, 84.5758) -> (-43.8244, 85.1092)
  line L280 (-43.8244, 85.1092) -> (-44.1801, 85.7494)
  line L281 (-44.1801, 85.7494) -> (-44.678, 86.7807)
  line L282 (-44.678, 86.7807) -> (-45.0336, 87.7054)
  line L283 (-45.0336, 87.7054) -> (-45.3537, 88.7368)
  line L284 (-45.3537, 88.7368) -> (-45.5671, 89.6614)
  line L285 (-45.5671, 89.6614) -> (-45.7449, 90.7284)
  line L286 (-45.7449, 90.7284) -> (-45.7805, 90.9773)
  line L287 (-45.7805, 90.9773) -> (-45.7805, 91.3685)
  line L288 (-34.8267, 96.9521) -> (-34.3643, 96.9521)
  line L289 (-34.3643, 96.9521) -> (-33.653, 96.881)
  line L290 (-33.653, 96.881) -> (-32.9062, 96.7032)
  line L291 (-32.9062, 96.7032) -> (-32.3727, 96.4898)
  line L292 (-32.3727, 96.4898) -> (-31.697, 96.1341)
  line L293 (-31.697, 96.1341) -> (-31.128, 95.7074)
  line L294 (-31.128, 95.7074) -> (-30.9146, 95.5295)
  line L295 (-30.9146, 95.5295) -> (-30.9146, 95.4584)
  line L296 (-30.9146, 95.4584) -> (-30.8435, 95.4584)
  line L297 (-30.8435, 95.4584) -> (-30.8435, 95.3873)
  line L298 (-30.8435, 95.3873) -> (-30.7723, 95.3873)
  line L299 (-30.7723, 95.3873) -> (-30.5234, 95.1028)
  line L300 (-30.5234, 95.1028) -> (-30.2389, 94.7471)
  line L301 (-30.2389, 94.7471) -> (-29.9188, 94.2137)
  line L302 (-29.9188, 94.2137) -> (-29.6698, 93.6802)
  line L303 (-29.6698, 93.6802) -> (-29.4565, 93.0401)
  line L304 (-29.4565, 93.0401) -> (-29.3142, 92.2221)
  line L305 (-29.3142, 92.2221) -> (-29.3142, 91.2618)
  line L306 (-29.3142, 91.2618) -> (-29.4209, 90.5506)
  line L307 (-29.4209, 90.5506) -> (-29.5987, 89.946)
  line L308 (-29.5987, 89.946) -> (-29.8121, 89.4125)
  line L309 (-29.8121, 89.4125) -> (-30.0966, 88.879)
  line L310 (-30.0966, 88.879) -> (-30.4167, 88.4523)
  line L311 (-30.4167, 88.4523) -> (-30.7368, 88.0966)
  line L312 (-30.7368, 88.0966) -> (-31.0924, 87.741)
  line L313 (-31.0924, 87.741) -> (-31.6614, 87.3142)
  line L314 (-31.6614, 87.3142) -> (-32.1593, 87.0297)
  line L315 (-32.1593, 87.0297) -> (-32.8706, 86.7452)
  line L316 (-32.8706, 86.7452) -> (-33.4397, 86.6029)
  line L317 (-33.4397, 86.6029) -> (-33.902, 86.5318)
  line L318 (-33.902, 86.5318) -> (-34.471, 86.4962)
  line L319 (-34.471, 86.4962) -> (-34.8978, 86.4962)
  line L320 (-34.8978, 86.4962) -> (-35.5735, 86.5674)
  line L321 (-35.5735, 86.5674) -> (-36.3204, 86.7452)
  line L322 (-36.3204, 86.7452) -> (-37.0317, 87.0297)
  line L323 (-37.0317, 87.0297) -> (-37.5295, 87.3142)
  line L324 (-37.5295, 87.3142) -> (-37.9208, 87.5987)
  line L325 (-37.9208, 87.5987) -> (-38.3831, 87.9899)
  line L326 (-38.3831, 87.9899) -> (-38.7743, 88.4167)
  line L327 (-38.7743, 88.4167) -> (-39.1655, 88.9857)
  line L328 (-39.1655, 88.9857) -> (-39.5211, 89.6614)
  line L329 (-39.5211, 89.6614) -> (-39.7345, 90.3016)
  line L330 (-39.7345, 90.3016) -> (-39.8768, 91.0129)
  line L331 (-39.8768, 91.0129) -> (-39.9124, 91.2974)
  line L332 (-39.9124, 91.2974) -> (-39.9124, 92.2576)
  line L333 (-39.9124, 92.2576) -> (-39.8057, 92.8978)
  line L334 (-39.8057, 92.8978) -> (-39.6278, 93.5024)
  line L335 (-39.6278, 93.5024) -> (-39.3433, 94.1425)
  line L336 (-39.3433, 94.1425) -> (-39.0232, 94.676)
  line L337 (-39.0232, 94.676) -> (-38.6676, 95.1383)
  line L338 (-38.6676, 95.1383) -> (-38.4187, 95.4229)
  line L339 (-38.4187, 95.4229) -> (-38.1341, 95.6718)
  line L340 (-38.1341, 95.6718) -> (-37.5651, 96.0986)
  line L341 (-37.5651, 96.0986) -> (-36.9961, 96.4187)
  line L342 (-36.9961, 96.4187) -> (-36.2848, 96.7032)
  line L343 (-36.2848, 96.7032) -> (-35.538, 96.881)
  line L344 (-35.538, 96.881) -> (-34.8267, 96.9521)
  line L345 (-30.1677, 100.0818) -> (-29.172, 100.0818)
  line L346 (-29.172, 100.0818) -> (-28.3895, 99.9395)
  line L347 (-28.3895, 99.9395) -> (-27.7849, 99.7617)
  line L348 (-27.7849, 99.7617) -> (-27.0737, 99.4416)
  line L349 (-27.0737, 99.4416) -> (-26.5046, 99.1215)
  line L350 (-26.5046, 99.1215) -> (-25.9356, 98.6948)
  line L351 (-25.9356, 98.6948) -> (-25.7222, 98.5169)
  line L352 (-25.7222, 98.5169) -> (-25.7222, 98.4458)
  line L353 (-25.7222, 98.4458) -> (-25.58, 98.3747)
  line L354 (-25.58, 98.3747) -> (-25.1532, 97.9124)
  line L355 (-25.1532, 97.9124) -> (-24.7975, 97.45)
  line L356 (-24.7975, 97.45) -> (-24.513, 96.9877)
  line L357 (-24.513, 96.9877) -> (-24.1218, 96.2408)
  line L358 (-24.1218, 96.2408) -> (-23.8373, 95.5295)
  line L359 (-23.8373, 95.5295) -> (-23.5884, 94.6404)
  line L360 (-23.5884, 94.6404) -> (-23.4461, 93.8936)
  line L361 (-23.4461, 93.8936) -> (-23.375, 93.2179)
  line L362 (-23.375, 93.2179) -> (-23.375, 92.0798)
  line L363 (-23.375, 92.0798) -> (-28.5674, 92.0443)
  line L364 (-28.5674, 92.0443) -> (-28.6385, 92.1865)
  line L365 (-28.6385, 92.1865) -> (-28.7452, 92.9334)
  line L366 (-28.7452, 92.9334) -> (-28.7452, 93.0756)
  line L367 (-28.7452, 93.0756) -> (-28.5674, 93.1112)
  line L368 (-28.5674, 93.1112) -> (-24.5486, 93.1467)
  line L369 (-24.5486, 93.1467) -> (-24.3708, 93.3246)
  line L370 (-24.3708, 93.3246) -> (-24.3708, 93.538)
  line L371 (-24.3708, 93.538) -> (-24.513, 93.7158)
  line L372 (-24.513, 93.7158) -> (-28.9586, 93.7513)
  line L373 (-28.9586, 93.7513) -> (-29.3853, 94.6049)
  line L374 (-29.3853, 94.6049) -> (-29.5276, 94.8538)
  line L375 (-29.5276, 94.8538) -> (-29.492, 94.9961)
  line L376 (-29.492, 94.9961) -> (-29.172, 95.2806)
  line L377 (-29.172, 95.2806) -> (-28.7807, 95.6007)
  line L378 (-28.7807, 95.6007) -> (-28.5318, 95.7785)
  line L379 (-28.5318, 95.7785) -> (-27.6071, 95.7785)
  line L380 (-27.6071, 95.7785) -> (-27.536, 95.5295)
  line L381 (-27.536, 95.5295) -> (-27.4293, 95.2095)
  line L382 (-27.4293, 95.2095) -> (-27.1804, 94.8894)
  line L383 (-27.1804, 94.8894) -> (-26.8247, 94.676)
  line L384 (-26.8247, 94.676) -> (-26.5402, 94.6049)
  line L385 (-26.5402, 94.6049) -> (-26.1134, 94.6049)
  line L386 (-26.1134, 94.6049) -> (-25.7222, 94.7471)
  line L387 (-25.7222, 94.7471) -> (-25.3666, 95.0672)
  line L388 (-25.3666, 95.0672) -> (-25.1888, 95.4584)
  line L389 (-25.1888, 95.4584) -> (-25.1532, 95.6362)
  line L390 (-25.1532, 95.6362) -> (-25.1532, 95.9563)
  line L391 (-25.1532, 95.9563) -> (-25.2954, 96.3831)
  line L392 (-25.2954, 96.3831) -> (-25.6155, 96.7387)
  line L393 (-25.6155, 96.7387) -> (-25.9712, 96.9166)
  line L394 (-25.9712, 96.9166) -> (-26.1134, 96.9521)
  line L395 (-26.1134, 96.9521) -> (-26.5758, 96.9521)
  line L396 (-26.5758, 96.9521) -> (-26.9314, 96.8454)
  line L397 (-26.9314, 96.8454) -> (-27.2515, 96.5965)
  line L398 (-27.2515, 96.5965) -> (-27.3582, 96.4542)
  line L399 (-27.3582, 96.4542) -> (-27.8205, 96.4187)
  line L400 (-27.8205, 96.4187) -> (-28.8519, 96.3831)
  line L401 (-28.8519, 96.3831) -> (-29.2786, 96.063)
  line L402 (-29.2786, 96.063) -> (-29.6698, 95.7074)
  line L403 (-29.6698, 95.7074) -> (-29.9188, 95.494)
  line L404 (-29.9188, 95.494) -> (-30.0255, 95.5295)
  line L405 (-30.0255, 95.5295) -> (-30.2744, 95.8141)
  line L406 (-30.2744, 95.8141) -> (-30.7368, 96.2764)
  line L407 (-30.7368, 96.2764) -> (-30.5234, 96.5253)
  line L408 (-30.5234, 96.5253) -> (-30.0966, 96.9166)
  line L409 (-30.0966, 96.9166) -> (-29.8832, 97.1299)
  line L410 (-29.8832, 97.1299) -> (-29.4209, 97.1299)
  line L411 (-29.4209, 97.1299) -> (-29.0653, 97.2366)
  line L412 (-29.0653, 97.2366) -> (-28.7807, 97.45)
  line L413 (-28.7807, 97.45) -> (-28.6385, 97.6278)
  line L414 (-28.6385, 97.6278) -> (-28.5318, 97.8768)
  line L415 (-28.5318, 97.8768) -> (-28.4962, 98.1969)
  line L416 (-28.4962, 98.1969) -> (-28.5674, 98.5169)
  line L417 (-28.5674, 98.5169) -> (-28.7096, 98.8015)
  line L418 (-28.7096, 98.8015) -> (-28.9941, 99.0504)
  line L419 (-28.9941, 99.0504) -> (-29.3498, 99.1927)
  line L420 (-29.3498, 99.1927) -> (-29.741, 99.1927)
  line L421 (-29.741, 99.1927) -> (-30.0611, 99.086)
  line L422 (-30.0611, 99.086) -> (-30.3811, 98.8015)
  line L423 (-30.3811, 98.8015) -> (-30.5234, 98.5169)
  line L424 (-30.5234, 98.5169) -> (-30.559, 98.3747)
  line L425 (-30.559, 98.3747) -> (-30.559, 97.9835)
  line L426 (-30.559, 97.9835) -> (-30.4167, 97.6278)
  line L427 (-30.4167, 97.6278) -> (-30.4523, 97.4856)
  line L428 (-30.4523, 97.4856) -> (-31.2347, 96.7032)
  line L429 (-31.2347, 96.7032) -> (-31.4125, 96.7387)
  line L430 (-31.4125, 96.7387) -> (-31.7681, 96.9877)
  line L431 (-31.7681, 96.9877) -> (-31.8037, 98.3747)
  line L432 (-31.8037, 98.3747) -> (-31.9104, 98.5881)
  line L433 (-31.9104, 98.5881) -> (-31.9815, 98.6236)
  line L434 (-31.9815, 98.6236) -> (-32.2305, 98.6236)
  line L435 (-32.2305, 98.6236) -> (-32.4083, 98.4458)
  line L436 (-32.4083, 98.4458) -> (-32.4439, 97.3078)
  line L437 (-32.4439, 97.3078) -> (-32.515, 97.2722)
  line L438 (-32.515, 97.2722) -> (-33.1196, 97.45)
  line L439 (-33.1196, 97.45) -> (-33.6886, 97.5567)
  line L440 (-33.6886, 97.5567) -> (-34.2576, 97.6278)
  line L441 (-34.2576, 97.6278) -> (-34.2576, 98.6236)
  line L442 (-34.2576, 98.6236) -> (-33.653, 98.837)
  line L443 (-33.653, 98.837) -> (-33.0485, 99.1571)
  line L444 (-33.0485, 99.1571) -> (-32.3727, 99.5127)
  line L445 (-32.3727, 99.5127) -> (-31.6614, 99.7973)
  line L446 (-31.6614, 99.7973) -> (-30.9857, 99.9751)
  line L447 (-30.9857, 99.9751) -> (-30.1677, 100.0818)
  line L448 (-39.9835, 100.0818) -> (-38.8454, 100.0818)
  line L449 (-38.8454, 100.0818) -> (-38.1697, 99.9751)
  line L450 (-38.1697, 99.9751) -> (-37.4584, 99.7617)
  line L451 (-37.4584, 99.7617) -> (-36.925, 99.5483)
  line L452 (-36.925, 99.5483) -> (-36.3559, 99.2638)
  line L453 (-36.3559, 99.2638) -> (-35.6446, 98.8726)
  line L454 (-35.6446, 98.8726) -> (-34.9334, 98.6236)
  line L455 (-34.9334, 98.6236) -> (-34.9334, 97.6278)
  line L456 (-34.9334, 97.6278) -> (-35.7513, 97.5211)
  line L457 (-35.7513, 97.5211) -> (-36.3559, 97.3789)
  line L458 (-36.3559, 97.3789) -> (-36.676, 97.2722)
  line L459 (-36.676, 97.2722) -> (-36.7827, 97.2722)
  line L460 (-36.7827, 97.2722) -> (-36.8183, 98.4103)
  line L461 (-36.8183, 98.4103) -> (-36.925, 98.5881)
  line L462 (-36.925, 98.5881) -> (-36.9961, 98.6236)
  line L463 (-36.9961, 98.6236) -> (-37.245, 98.6236)
  line L464 (-37.245, 98.6236) -> (-37.3873, 98.5169)
  line L465 (-37.3873, 98.5169) -> (-37.4229, 98.4103)
  line L466 (-37.4229, 98.4103) -> (-37.4584, 96.9877)
  line L467 (-37.4584, 96.9877) -> (-37.8496, 96.7032)